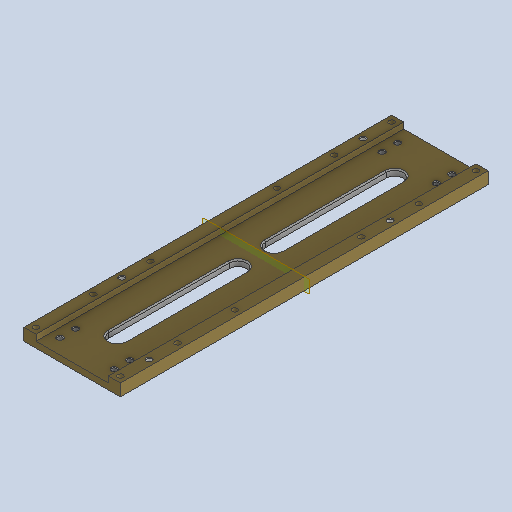
# Autodesk Inventor part: TS_V1_Fallmagazin_Boden_int
Saved by Autodesk Inventor 2025.2 (Build 292293000, 293)
## iProperties
Created: 2025-06-10
Part Number: TS_V1_Fallmagazin_Boden_int
Material: Generisch
Document SubType Name: Modeling
Designer: tino
Density: 1 g/cm^3
Appearance: Vorgabe
Author: tino
Autodesk Inventor part; units mm, degrees
ref_plane "YZ Plane" through (0, 0, 0) normal (1, 0, 0) x (0, 1, 0)
ref_plane "XY Plane" through (0, 0, 0) normal (0, 0, 1) x (1, 0, 0)
sketch "Skizze1" plane through (0, 0, 0) normal (0, 0, 1) x (1, 0, 0)
  line L0 (-40, 152.5) -> (40, 152.5)
  line L1 (40, 152.5) -> (40, -152.5)
  line L2 (40, -152.5) -> (-40, -152.5)
  line L3 (-40, -152.5) -> (-40, 152.5)
  line L4 (-40, 152.5) -> (40, -152.5) construction
  line L5 (40, 152.5) -> (-40, -152.5) construction
  point P0 (0, 0)
  dimension "d2" = 80
  dimension "d3" = 305
  constraints: 12 end point, 2 midpoint, 2 parallel, 1 horizontal, 1 perpendicular
  measures "d2" distance of L0.start L0.end
  measures "d3" distance of L2.end L0.start
extrude "Extrusion1" add sketch "Skizze1" along normal blind 10
sketch "Skizze2" plane through (0, 0, 0) normal (0, 0, -1) x (-1, 0, 0)
  point P0 (0, 0)
  point P1 (-35, 147.5)
  dimension "d6" = 147.5
  dimension "d7" = 35
  measures "d6" vertical distance of point (0, 0) point (-35, 147.5)
  measures "d7" horizontal distance of point (0, 0) point (-35, 147.5)
sketch "Skizze4" plane through (0, 0, 10) normal (0, 0, 1) x (1, 0, 0)
  spline S0 degree 3 poles (4.1682, 35.1897) (1.1905, 36.4598) (-2.2497, 35.1642) (-6.2549, 34.1582) (-11.736, 32.1479) (-17.2675, 27.437) (-17.3979, 22.2805) (-19.1794, 11.8373) (-24.2043, -4.2198) (-21.9122, -21.3618) (-15.7263, -32.1361) (-8.9601, -34.8731) (-7.7344, -35.2068) knots 0 0 0 0 0.05535 0.076528 0.211782 0.295547 0.382964 0.432922 0.754884 0.81234 0.967238 1 1 1 1
  spline S1 degree 3 poles (-7.7344, -35.2068) (-2.4391, -36.6482) (4.9342, -35.145) (14.3889, -31.3641) (20.2206, -28.2766) (23.0847, -23.1792) (23.281, -18.9959) (17.3062, -16.4997) (13.7398, -19.2937) (6.9074, -22.9332) (-1.1986, -27.1621) (-10.3055, -22.9326) (-14.0352, -10.4002) (-9.4599, -0.926) (-6.8333, 0.3153) (-5.9182, 2.0588) (-5.9367, 4.1791) (-8.2887, 5.2306) (-8.3641, 10.4373) (-1.0106, 14.1251) (4.0821, 20.0507) (3.0635, 26.3026) (2.9493, 28.6136) (3.7888, 29.834) (5.5778, 31.0924) (6.6132, 32.7745) (5.2458, 34.7086) (4.2657, 35.1481) (4.1682, 35.1897) knots 0 0 0 0 0.14153 0.17035 0.245987 0.25892 0.290227 0.326265 0.372233 0.38898 0.482096 0.508256 0.624416 0.647418 0.715274 0.72607 0.746892 0.801722 0.811885 0.848514 0.916356 0.943374 0.948219 0.962959 0.96651 0.98188 0.998188 1 1 1 1
  arc A0 (-7.9107, 24.207) -> (-7.9109, 20.407) centre (-6.0635, 22.307) ccw
  line L0 (-7.9107, 24.207) -> (-4.2161, 24.2069)
  arc A1 (-4.2163, 20.4069) -> (-4.2161, 24.2069) centre (-6.0635, 22.307) ccw
  line L1 (-4.2163, 20.4069) -> (-7.9109, 20.407)
  spline S2 degree 3 poles (4.1682, 35.1897) (1.1905, 36.4598) (-2.2497, 35.1642) (-6.255, 34.1582) (-11.7361, 32.1479) (-17.2675, 27.437) (-17.3979, 22.2805) (-19.1794, 11.8373) (-24.2043, -4.2198) (-21.9122, -21.3619) (-15.7263, -32.1361) (-8.9601, -34.8731) (-7.7344, -35.2068) knots 0 0 0 0 0.05535 0.076528 0.211782 0.295547 0.382964 0.432922 0.754884 0.81234 0.967238 1 1 1 1
  spline S3 degree 3 poles (-7.7344, -35.2068) (-2.4391, -36.6482) (4.9342, -35.145) (14.3889, -31.3641) (20.2206, -28.2766) (23.0847, -23.1792) (23.281, -18.9959) (17.3062, -16.4997) (13.7398, -19.2937) (6.9074, -22.9332) (-1.1986, -27.1621) (-10.3055, -22.9326) (-14.0352, -10.4002) (-9.4599, -0.926) (-6.8333, 0.3153) (-5.9182, 2.0588) (-5.9367, 4.1791) (-8.2887, 5.2306) (-8.3641, 10.4373) (-1.0106, 14.1251) (4.0821, 20.0507) (3.0635, 26.3026) (2.9493, 28.6136) (3.7888, 29.834) (5.5778, 31.0924) (6.6132, 32.7745) (5.2458, 34.7086) (4.2657, 35.1481) (4.1682, 35.1897) knots 0 0 0 0 0.14153 0.17035 0.245987 0.25892 0.290227 0.326265 0.372233 0.38898 0.482096 0.508256 0.624416 0.647418 0.715274 0.72607 0.746892 0.801722 0.811885 0.848514 0.916356 0.943374 0.948219 0.962959 0.96651 0.98188 0.998188 1 1 1 1
  line L2 (-4.2163, 20.4069) -> (-7.9109, 20.407)
  arc A2 (-4.2163, 20.4069) -> (-4.2161, 24.2069) centre (-6.0635, 22.307) ccw
  line L3 (-7.9107, 24.207) -> (-4.2161, 24.2069)
  arc A3 (-7.9107, 24.207) -> (-7.9109, 20.407) centre (-6.0635, 22.307) ccw
  line L4 (-22.9949, 35.8296) -> (22.9949, 35.8296) construction
  line L5 (22.9949, 35.8296) -> (22.9949, -35.8296) construction
  line L6 (22.9949, -35.8296) -> (-22.9949, -35.8296) construction
  line L7 (-22.9949, -35.8296) -> (-22.9949, 35.8296) construction
  line L8 (-22.9949, 35.8296) -> (22.9949, -35.8296) construction
  line L9 (-22.9949, -35.8296) -> (22.9949, 35.8296) construction
  point P0 (0, 0)
  point P1 (0, 0)
  point P2 (0, 0)
  constraints: 20 end point, 8 point on circle, 4 centre point, 3 horizontal, 3 perpendicular, 2 vertical, 1 midpoint, 8 other
hole "Bohrung2" at (35, 147.5, 0) direction (0, 0, 1) diameter 4.5 end through all counterbore diameter 8 counterbore depth 4.4
pattern_linear "Rechteckige Anordnung2" count 3 spacing 47.5 along (0, -1, 0) count 2 spacing 70 along (-1, 0, 0) of "Bohrung2"
mirror "Spiegeln2" about plane through (0, 0, 0) normal (0, 1, 0) of "Bohrung2", "Rechteckige Anordnung2"
sketch "Skizze7" plane through (0, 0, 10) normal (0, 0, 1) x (1, 0, 0)
  line L0 (-40, -152.5) -> (40, -152.5) projected
  line L1 (-30, 152.5) -> (30, 152.5)
  line L2 (30, 152.5) -> (30, -152.5)
  line L3 (30, -152.5) -> (-30, -152.5)
  line L4 (-30, -152.5) -> (-30, 152.5)
  line L5 (-40, 152.5) -> (-40, -152.5) projected
  line L6 (40, 152.5) -> (-40, 152.5) projected
  point P0 (0, 0)
  dimension "d99" = 60
  dimension "d100" = 10
  constraints: 8 end point, 2 parallel, 1 collinear, 1 horizontal, 1 perpendicular, 1 point on line
  measures "d99" distance between parallel lines of L2 L4
  measures "d100" distance between parallel lines of L4 L5
extrude "Extrusion4" cut sketch "Skizze7" against normal blind 5 contours L4 L1 L2 L0
sketch "Skizze8" plane through (0, 0, 5) normal (0, 0, 1) x (1, 0, 0)
  arc A0 (-32.75, -100) -> (-32.75, -100) centre (-35, -100) ccw projected
  arc A1 (37.25, -100) -> (37.25, -100) centre (35, -100) ccw projected
  arc A2 (31, 100) -> (31, 100) centre (35, 100) ccw projected
  arc A3 (-32.75, 100) -> (-32.75, 100) centre (-35, 100) ccw projected
  arc A4 (37.25, 100) -> (37.25, 100) centre (35, 100) ccw projected
  line L0 (30, -152.5) -> (-30, -152.5) projected
  line L1 (30, 152.5) -> (30, -152.5) projected
  line L2 (-30, 152.5) -> (30, 152.5) projected
  line L3 (-30, -152.5) -> (-30, 152.5) projected
  line L4 (-7, -122) -> (7, -122)
  line L5 (7, -122) -> (7, -8)
  line L6 (7, -8) -> (-7, -8)
  line L7 (-7, -8) -> (-7, -122)
  arc A5 (31, -100) -> (31, -100) centre (35, -100) ccw construction
  line L8 (-35, -100) -> (35, -100) construction
  arc A6 (-39, 100) -> (-39, 100) centre (-35, 100) ccw construction
  line L9 (-35, 100) -> (35, 100) construction
  arc A7 (7, -15) -> (-7, -15) centre (0, -15) ccw
  arc A8 (-7, -115) -> (7, -115) centre (0, -115) ccw
  line L10 (-68.4872, 0) -> (66.5847, 0) projected
  line L11 (-7, 122) -> (7, 122)
  line L12 (7, 122) -> (7, 8)
  line L13 (7, 8) -> (-7, 8)
  line L14 (-7, 8) -> (-7, 122)
  arc A9 (-7, 15) -> (7, 15) centre (0, 15) ccw
  arc A10 (7, 115) -> (-7, 115) centre (0, 115) ccw
  line L15 (-49.1912, -115) -> (47.2887, -115) construction
  point P0 (0, 0)
  dimension "d105" = 14
  dimension "d106" = 7
  dimension "d114" = 15
  dimension "d115" = 100
  constraints: 22 end point, 10 symmetric about line, 9 point on line, 8 point on circle, 6 tangent, 4 centre point, 4 horizontal, 2 parallel, 1 perpendicular, 2 other
  measures "d105" distance of L4.start L4.end
  measures "d106" distance from line of L5 point (0, 0)
  measures "d114" distance from line of L15 L8.start
  measures "d115" distance of A8.centre A7.centre
extrude "Extrusion5" cut sketch "Skizze8" against normal through all contours A8 L7 A7 L5 | A10 L12 A9 L14
sketch "Skizze9" plane through (0, 0, 5) normal (0, 0, 1) x (1, 0, 0)
  line L0 (30, -152.5) -> (-30, -152.5) projected
  point P0 (0, 0)
  point P1 (-22.5, -140.1)
  point P2 (0, -152.5)
  dimension "d116" = 22.5
  dimension "d117" = 12.4
  constraints: 1 midpoint
  measures "d116" horizontal distance of point (0, -152.5) point (-22.5, -140.1)
  measures "d117" distance from line of L0 point (-22.5, -140.1)
hole "Bohrung3" at (-22.5, -140.1, 5) direction (0, 0, -1) diameter 4.134 end through all thread size "M5x0.8" class "6H" standard "ISO Metric profile"
chamfer "Fasen2" distance 0.5 angle 45 2 edges at (-22.5, -138.033, 5) (-22.5, -138.033, 0)
pattern_linear "Rechteckige Anordnung3" count 2 spacing 45 along (1, 0, 0) count 2 spacing 13 along (0, 1, 0) of "Bohrung3", "Fasen2"
mirror "Spiegeln3" about plane through (0, 0, 0) normal (0, 1, 0) of "Bohrung3", "Fasen2", "Rechteckige Anordnung3"
sketch "Skizze10" plane through (0, 0, 10) normal (0, 0, 1) x (1, 0, 0)
  circle A0 centre (35, -147.5) radius 2.25 projected
  circle A1 centre (-35, -52.5) radius 2.25 projected
  circle A2 centre (-35, -100) radius 2.25 projected
  circle A3 centre (35, -100) radius 2.25 projected
  circle A4 centre (35, 100) radius 2.25 projected
  circle A5 centre (35, 147.5) radius 2.25 projected
  circle A6 centre (-35, 100) radius 2.25 projected
  circle A7 centre (-35, 52.5) radius 2.25 projected
  point P0 (0, 0)
  point P1 (35, -123.75)
  point P2 (-35, -76.25)
  point P3 (-35, 123.75)
  point P4 (35, 76.25)
  dimension "d137" = 23.75
  dimension "d138" = 23.75
  dimension "d149" = 23.75
  dimension "d150" = 23.75
  constraints: 4 vertical alignment
  measures "d137" distance of A1.centre point (-35, -76.25)
  measures "d138" distance of A0.centre point (35, -123.75)
  measures "d149" distance of A6.centre point (-35, 123.75)
  measures "d150" distance of A4.centre point (35, 76.25)
hole "Bohrung4" at (35, -123.75, 10) at (-35, -76.25, 10) at (-35, 123.75, 10) at (35, 76.25, 10) direction (0, 0, -1) diameter 4 depth 5.5 countersink diameter 5 countersink angle 90
chamfer "Fasen3" distance 1 angle 45 8 edges at (-7, 65, 5) (0, 122, 5) (7, 65, 5) (0, 8, 5) (-7, -65, 5) (0, -8, 5) (7, -65, 5) (0, -122, 5)
equation "\"d2\" = Breite_aussen"
equation "\"d3\" = 2 * Laenge_aussen + Zwischenteil"
equation "\"d4\" = Wanddicke"
equation "\"d6\" = 0.5 * Zwischenteil + Laenge_aussen - 0.5 * Wanddicke"
equation "\"d7\" = -0.5 * Wanddicke + 0.5 * Breite_aussen"
equation "\"d95\" = -0.5 * Wanddicke + 0.5 * Laenge_aussen"
equation "\"d98\" = Breite_aussen - Wanddicke"
equation "\"d99\" = Breite_aussen - 2 * Wanddicke"
equation "\"d100\" = Wanddicke"
equation "\"d101\" = Absatz"
equation "\"d105\" = Kolbenanbindung_Breite"
equation "\"d106\" = 0.5 * d105"
equation "\"d115\" = Kolbenhub"
equation "\"d137\" = d135"
equation "\"d138\" = d135"
equation "\"d149\" = d135"
equation "\"d150\" = d149"
equation "\"Breite_aussen\" = 80"
equation "\"Laenge_aussen\" = 105"
equation "\"Wanddicke\" = 10"
equation "\"Laenge_innen\" = Laenge_aussen - Wanddicke"
equation "\"Absatz\" = 5"
equation "\"Kolbenhub\" = 100"
equation "\"Kolbenanbindung_Breite\" = 14"
equation "\"d135\" = 0.5 * d134"
equation "\"Zwischenteil\" = 95"
equation "\"d134\" = 47.5"
